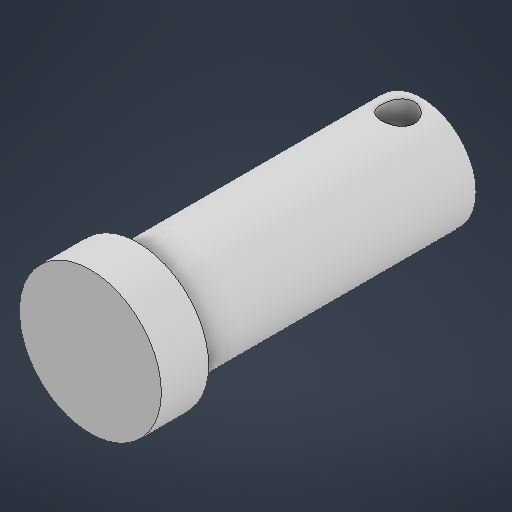
# Autodesk Inventor part: Pin
Saved by Autodesk Inventor 2026.1 (Build 301233020, 233B)
## iProperties
Created: 2025-10-06
Part Number: Pin
Material: Generic
Document SubType Name: Modeling
Designer: Gamec
Density: 1 g/cm^3
Appearance: Default
Author: Gamec
Autodesk Inventor part; units mm, degrees
ref_plane "YZ Plane" through (0, 0, 0) normal (1, 0, 0) x (0, 1, 0)
ref_plane "XZ Plane" through (0, 0, 0) normal (0, 1, 0) x (-1, 0, 0)
sketch "Sketch1" plane through (0, 0, 0) normal (0, 0, 1) x (1, 0, 0)
  circle A0 centre (0, 0) radius 2.921
  dimension "d0" = 5.842
  constraints: 1 centre point, 1 coincident
  measures "d0" diameter of A0
extrude "Extrusion1" add sketch "Sketch1" along normal blind 12.7
sketch "Sketch2" plane through (0, 0, 12.7) normal (0, 0, 1) x (1, 0, 0)
  circle A0 centre (0, 0) radius 3.81
  dimension "d3" = 7.62
  constraints: 1 centre point, 1 coincident
  measures "d3" diameter of A0
extrude "Extrusion2" add sketch "Sketch2" along normal blind 2.54
sketch "Sketch3" plane through (0, 0, 0) normal (0, 0, -1) x (-1, 0, 0)
  circle A0 centre (0, 0) radius 2.921
  dimension "d12" = 5.842
  constraints: 1 centre point, 1 coincident
  measures "d12" diameter of A0
extrude "Extrusion3" add sketch "Sketch3" along normal blind 2.54
sketch "Sketch4" plane through (0, 0, -2.54) normal (0, 0, -1) x (-1, 0, 0)
  circle A0 centre (0, 0) radius 2.921 projected
  point P0 (0, 2.921)
  constraints: 1 vertical alignment, 1 other
ref_plane "Work Plane1" through (0, 2.921, -2.54) normal (0, 1, 0) x (-1, 0, 0)
sketch "Sketch5" plane through (0, 2.921, -2.54) normal (0, 1, 0) x (-1, 0, 0)
  circle A0 centre (0, 1.27) radius 0.885
  line L0 (-2.921, 0) -> (2.921, 0) projected
  point P0 (0, 2.54)
  dimension "d8" = 1.77
  dimension "d9" = 1.27
  constraints: 1 centre point
  measures "d8" diameter of A0
  measures "d9" distance from line of L0 A0.centre
extrude "Extrusion4" cut sketch "Sketch5" against normal blind 7.3025
body "Solid1"
